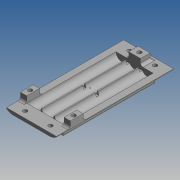
# Autodesk Inventor part: P040_BoitierCouvercleV4_module
Saved by Autodesk Inventor 2021.3 (Build 253353000, 353)
## iProperties
Created: 2021-12-17
Part Number: P040_BoitierCouvercleV4_module
Material: Générique
Document SubType Name: Modeling
Designer: gabri
Density: 1 g/cm^3
Appearance: Par défaut
Author: gabri
Autodesk Inventor part; units mm, degrees
note: some values were not read from the file. Chosen so that the rebuilt part matches the saved one: direction of "Hole1".
ref_plane "YZ Plane" through (0, 0, 0) normal (1, 0, 0) x (0, 1, 0)
ref_plane "XZ Plane" through (0, 0, 0) normal (0, 1, 0) x (-1, 0, 0)
sketch "Sketch2" plane through (0, 0, 0) normal (0, 0, 1) x (1, 0, 0)
  line L0 (30, -92) -> (-30, -92)
  line L1 (-30, -92) -> (-30, 92)
  line L2 (-30, 92) -> (30, 92)
  line L3 (30, 92) -> (30, -92)
  line L4 (30, -92) -> (-30, 92) construction
  line L5 (-30, -92) -> (30, 92) construction
  point P0 (0, 0)
  dimension "d0" = 60
  dimension "d1" = 184
  constraints: 12 end point, 2 midpoint, 2 parallel, 1 horizontal, 1 perpendicular
  measures "d0" distance between parallel lines of L3 L1
  measures "d1" distance between parallel lines of L0 L2
extrude "Extrusion1" add sketch "Sketch2" along normal blind 5
sketch "Sketch3" plane through (0, 0, 5) normal (0, 0, 1) x (1, 0, 0)
  line L0 (-30, -92) -> (30, -92) construction
  line L1 (30, 92) -> (-30, 92) construction
  line L2 (30, -92) -> (30, 92) construction
  line L3 (-30, 92) -> (-30, -92) construction
  point P0 (0, 0)
  point P1 (-20, 82)
  point P2 (20, 82)
  point P3 (-20, -82)
  point P4 (20, -82)
  dimension "d4" = 40
  dimension "d5" = 164
  dimension "d6" = 184
  dimension "d7" = 60
  dimension "d8" = 10
  dimension "d9" = 10
  dimension "d10" = 10
  dimension "d11" = 164
  dimension "d12" = 40
  dimension "d13" = 10
  measures "d4" distance of point (20, 82) point (-20, 82)
  measures "d5" distance of point (-20, 82) point (-20, -82)
  measures "d6" distance between parallel lines of L0 L1
  measures "d7" distance between parallel lines of L2 L3
  measures "d8" distance from line of L3 point (-20, 82)
  measures "d9" distance from line of L1 point (-20, 82)
  measures "d10" distance from line of L1 point (20, 82)
  measures "d11" distance of point (20, -82) point (20, 82)
  measures "d12" distance of point (20, -82) point (-20, -82)
  measures "d13" distance from line of L3 point (-20, -82)
hole "Hole1" at (-20, 82, 5) at (20, 82, 5) at (-20, -82, 5) at (20, -82, 5) direction (0, 0, -1) diameter 6.4 depth 5
sketch "Sketch4" plane through (0, 0, 5) normal (0, 0, 1) x (1, 0, 0)
  line L0 (-13.7576, 88.5859) -> (-6.8739, 88.5859) construction
  line L1 (-6.8739, 88.5859) -> (-6.8739, 84.2378) construction
  line L2 (-6.8739, 84.2378) -> (-13.7576, 84.2378) construction
  line L3 (-13.7576, 84.2378) -> (-13.7576, 88.5859) construction
  point P0 (0, 0)
  constraints: 2 other
sketch "Sketch5" plane through (0, 0, 5) normal (0, 0, 1) x (1, 0, 0)
  line L0 (-30, -72) -> (30, -72)
  line L1 (30, -72) -> (30, 72)
  line L2 (30, 72) -> (-30, 72)
  line L3 (-30, 72) -> (-30, -72)
  line L4 (-30, -72) -> (30, 72) construction
  line L5 (30, -72) -> (-30, 72) construction
  circle A0 centre (-20, -82) radius 3.2 construction
  circle A1 centre (-20, 82) radius 3.2 construction
  circle A2 centre (20, 82) radius 3.2 construction
  circle A3 centre (20, -82) radius 3.2 construction
  line L6 (30, 92) -> (-30, 92) construction
  line L7 (-30, 92) -> (-30, -92) construction
  line L8 (-30, -92) -> (30, -92) construction
  line L9 (30, -92) -> (30, 92) construction
  point P0 (0, 0)
  point P1 (30, 0)
  dimension "d21" = 10
  constraints: 12 end point, 4 midpoint, 2 parallel, 1 horizontal, 1 perpendicular
  measures "d21" distance from line of A2.centre L2
extrude "Extrusion2" add sketch "Sketch5" against normal blind 15
sketch "Sketch6" plane through (0, 0, 0) normal (0, 1, 0) x (-1, 0, 0)
  line L0 (-30, 5) -> (30, 5) construction
  line L1 (30, -10) -> (-30, -10) construction
  line L2 (30, 0) -> (30, 5) construction
  line L3 (-30, 0) -> (-30, 5) construction
  circle A0 centre (0, 5) radius 9.25
  circle A1 centre (-20, 5) radius 9.25
  line L4 (0, -13.85) -> (0, 20.1) construction
  circle A2 centre (20, 5) radius 9.25
  point P0 (0, 0)
  dimension "d24" = 18.5
  dimension "d27" = 18.5
  dimension "d40" = 18.5
  dimension "d41" = 20
  dimension "d42" = 20
  constraints: 4 point on line, 3 centre point, 2 midpoint
  measures "d24" diameter of A0
  measures "d27" diameter of A1
  measures "d40" diameter of A2
  measures "d41" distance of A0.centre A2.centre
  measures "d42" distance from line of L4 A1.centre
extrude "Extrusion3" cut sketch "Sketch6" along normal mid plane 140
fillet "Fillet2" radius 6 2 edges at (0, 72, 0) (0, -72, 0)
ref_plane "Work Plane1" through (0, 0, 4) normal (0, 0, -1) x (-1, 0, 0)
sketch "Sketch9" plane through (0, 0, 4) normal (0, 0, -1) x (-1, 0, 0)
  line L0 (30, -72) -> (30, 72) construction
  line L1 (30, 78) -> (-30, 78) construction
  line L2 (30, 92) -> (30, 78) construction
  line L3 (-30, 92) -> (30, 92) construction
  line L4 (-30, 78) -> (-30, 92) construction
  circle A0 centre (20, 82) radius 3.2 construction
  circle A1 centre (-20, 82) radius 3.2 construction
  line L5 (-30, 78) -> (-30, 72) construction
  line L6 (-30, 72) -> (30, 72) construction
  line L7 (30, 72) -> (30, 78) construction
  line L8 (30, 78) -> (-30, 78) construction
  line L9 (-30, -78) -> (30, -78) construction
  line L10 (-30, -92) -> (-30, -78) construction
  line L11 (30, -92) -> (-30, -92) construction
  line L12 (30, -78) -> (30, -92) construction
  circle A2 centre (20, -82) radius 3.2 construction
  circle A3 centre (-20, -82) radius 3.2 construction
  line L13 (30, -72) -> (-30, -72) construction
  line L14 (30, -78) -> (30, -72) construction
  line L15 (30, -72) -> (-30, -72) construction
  line L16 (-30, -72) -> (-30, -78) construction
  line L17 (-30, -78) -> (30, -78) construction
  line L18 (-30, 92) -> (-39.25, 92)
  line L19 (-39.25, 92) -> (-39.25, -92)
  line L20 (-39.25, -92) -> (-30, -92)
  line L21 (-30, -92) -> (-30, 92)
  line L22 (30, 92) -> (39.25, 92)
  line L23 (39.25, 92) -> (39.25, -92)
  line L24 (39.25, -92) -> (30, -92)
  line L25 (30, -92) -> (30, 92)
  point P0 (0, 0)
  dimension "d44" = 9.25
  dimension "d45" = 184
  dimension "d46" = 9.25
  dimension "d47" = 184
  constraints: 16 end point, 4 parallel, 2 horizontal, 2 perpendicular
  measures "d44" distance between parallel lines of L4 L19
  measures "d45" distance between parallel lines of L20 L18
  measures "d46" distance between parallel lines of L23 L2
  measures "d47" distance between parallel lines of L22 L24
extrude "Extrusion5" add sketch "Sketch9" against normal blind 1
sketch "Sketch10" plane through (0, 0, 5) normal (0, 0, 1) x (1, 0, 0)
  line L0 (9.25, -70) -> (-9.25, -70) construction
  line L1 (-9.25, -70) -> (-9.25, 70) construction
  line L2 (-9.25, 70) -> (9.25, 70) construction
  line L3 (9.25, 70) -> (9.25, -70) construction
  line L4 (29.25, -70) -> (10.75, -70) construction
  line L5 (10.75, -70) -> (10.75, 70) construction
  line L6 (10.75, 70) -> (29.25, 70) construction
  line L7 (29.25, 70) -> (29.25, -70) construction
  line L8 (-10.75, -70) -> (-29.25, -70) construction
  line L9 (-29.25, -70) -> (-29.25, 70) construction
  line L10 (-29.25, 70) -> (-10.75, 70) construction
  line L11 (-10.75, 70) -> (-10.75, -70) construction
  circle A0 centre (20, -82) radius 3.2 construction
  circle A1 centre (-20, -82) radius 3.2 construction
  line L12 (39.25, 92) -> (-39.25, 92) construction
  line L13 (-39.25, 92) -> (-39.25, -92) construction
  line L14 (-39.25, -92) -> (39.25, -92) construction
  line L15 (39.25, -92) -> (39.25, 92) construction
  circle A2 centre (20, 82) radius 3.2 construction
  circle A3 centre (-20, 82) radius 3.2 construction
  line L16 (29.25, -70) -> (39.25, -70)
  line L17 (39.25, -70) -> (39.25, -50)
  line L18 (39.25, -50) -> (29.25, -50)
  line L19 (29.25, -50) -> (29.25, -70)
  line L20 (-29.25, -70) -> (-39.25, -70)
  line L21 (-39.25, -70) -> (-39.25, -50)
  line L22 (-39.25, -50) -> (-29.25, -50)
  line L23 (-29.25, -50) -> (-29.25, -70)
  line L24 (9.25, 85) -> (-9.25, 85)
  line L25 (-9.25, 85) -> (-9.25, 70)
  line L26 (-9.25, 70) -> (9.25, 70)
  line L27 (9.25, 70) -> (9.25, 85)
  point P0 (0, 0)
  dimension "d55" = 10
  dimension "d56" = 10
  dimension "d57" = 20
  dimension "d58" = 15
  dimension "d59" = 18.5
  constraints: 24 end point, 6 parallel, 3 horizontal, 3 perpendicular, 1 point on line
  measures "d55" distance between parallel lines of L7 L17
  measures "d56" distance between parallel lines of L21 L23
  measures "d57" distance between parallel lines of L16 L18
  measures "d58" distance between parallel lines of L2 L24
  measures "d59" distance between parallel lines of L25 L27
extrude "Extrusion6" add sketch "Sketch10" along normal blind 10
fillet "Fillet6" radius 4 7 edges at (34.25, -50, 5) (34.25, -70, 5) (-34.25, -70, 5) (-34.25, -50, 5) (9.25, 77.5, 5) (0, 85, 5) (-9.25, 77.5, 5)
sketch "Sketch11" plane through (-30, 92, 0) normal (0, 1, 0) x (1, 0, 0)
  line L0 (60, 0) -> (0, 0) construction
  line L1 (0, 0) -> (0, -4) construction
  line L2 (-9.25, -4) -> (0, -4) construction
  line L3 (-9.25, -4) -> (-9.25, -5) construction
  line L4 (69.25, -5) -> (-9.25, -5) construction
  line L5 (69.25, -4) -> (69.25, -5) construction
  line L6 (60, -4) -> (69.25, -4) construction
  line L7 (60, 0) -> (60, -4) construction
  line L8 (69.25, -4) -> (60, -4)
  line L9 (0, 0) -> (0, -4)
  line L10 (0, -4) -> (-9.25, -4)
  line L11 (60, -4) -> (60, 0)
  arc A0 (0, 0) -> (-9.25, -4) centre (0.9827, -14.9678) ccw
  arc A1 (69.25, -4) -> (60, 0) centre (56.9429, -19.765) ccw
  point P0 (30, 0)
  dimension "d68" = 15
  dimension "d69" = 20
  constraints: 8 end point, 4 point on circle, 3 collinear, 2 centre point, 1 perpendicular
  measures "d68" radius of A0
  measures "d69" radius of A1
extrude "Extrusion7" add sketch "Sketch11" against normal up to surface (184 mm away)
fillet "Fillet7" radius 2 4 edges at (0, 72, -10) (-30, 0, -10) (0, -72, -10) (30, 0, -10)
sketch "Sketch12" plane through (0, 0, 15) normal (0, 0, 1) x (1, 0, 0)
  line L0 (0, 128.8) -> (0, -128.8) construction
  line L1 (-9.25, 85) -> (-9.25, 70) construction
  line L2 (-9.25, 70) -> (9.25, 70) construction
  line L3 (9.25, 70) -> (9.25, 85) construction
  line L4 (9.25, 85) -> (-9.25, 85) construction
  line L5 (39.25, -70) -> (39.25, -50) construction
  line L6 (39.25, -50) -> (29.25, -50) construction
  line L7 (29.25, -50) -> (29.25, -70) construction
  line L8 (29.25, -70) -> (39.25, -70) construction
  line L9 (-29.25, -50) -> (-39.25, -50) construction
  line L10 (-39.25, -50) -> (-39.25, -70) construction
  line L11 (-39.25, -70) -> (-29.25, -70) construction
  line L12 (-29.25, -70) -> (-29.25, -50) construction
  point P0 (0, 0)
  point P1 (0, 77.5)
  point P2 (-34.25, -60)
  point P3 (34.25, -60)
  dimension "d70" = 9.25
  dimension "d71" = 7.5
  dimension "d102" = 5
  dimension "d103" = 5
  dimension "d104" = 10
  dimension "d105" = 10
  constraints: 1 point on line
  measures "d70" distance from line of L3 point (0, 77.5)
  measures "d71" distance from line of L2 point (0, 77.5)
  measures "d102" distance from line of L12 point (-34.25, -60)
  measures "d103" distance from line of L5 point (34.25, -60)
  measures "d104" distance from line of L11 point (-34.25, -60)
  measures "d105" distance from line of L8 point (34.25, -60)
hole "Hole2" at (0, 77.5, 15) at (34.25, -60, 15) at (-34.25, -60, 15) direction (0, 0, -1) diameter 6.4 depth 9.5
sketch "Sketch13" plane through (0, 0, 5) normal (0, 0, 1) x (1, 0, 0)
  line L0 (-29.25, -70) -> (-29.25, -46) construction
  line L1 (-29.25, -70) -> (-10.75, -70) construction
  line L2 (-10.75, 70) -> (-10.75, -70) construction
  line L3 (-10.75, 70) -> (-29.25, 70) construction
  line L4 (-29.25, -46) -> (-29.25, 70) construction
  line L5 (-9.25, -70) -> (-9.25, 70) construction
  line L6 (-9.25, -70) -> (9.25, -70) construction
  line L7 (9.25, 70) -> (9.25, -70) construction
  line L8 (9.25, 70) -> (-9.25, 70) construction
  line L9 (10.75, -70) -> (10.75, 70) construction
  line L10 (10.75, -70) -> (29.25, -70) construction
  line L11 (29.25, -46) -> (29.25, -70) construction
  line L12 (29.25, 70) -> (29.25, -46) construction
  line L13 (29.25, 70) -> (10.75, 70) construction
  line L14 (-12.75, -70) -> (-7.25, -70)
  line L15 (-7.25, -70) -> (-7.25, -66)
  line L16 (-7.25, -66) -> (-12.75, -66)
  line L17 (-12.75, -66) -> (-12.75, -70)
  line L18 (7.25, -66) -> (7.25, -70)
  line L19 (7.25, -70) -> (12.75, -70)
  line L20 (12.75, -66) -> (7.25, -66)
  line L21 (12.75, -70) -> (12.75, -66)
  line L22 (-12.75, 2) -> (-12.75, -2)
  line L23 (-12.75, -2) -> (-7.25, -2)
  line L24 (-7.25, 2) -> (-12.75, 2)
  line L25 (-7.25, -2) -> (-7.25, 2)
  line L26 (7.25, 2) -> (7.25, -2)
  line L27 (7.25, -2) -> (12.75, -2)
  line L28 (12.75, 2) -> (7.25, 2)
  line L29 (12.75, -2) -> (12.75, 2)
  line L30 (-12.75, 70) -> (-12.75, 66)
  line L31 (-12.75, 66) -> (-7.25, 66)
  line L32 (-7.25, 70) -> (-12.75, 70)
  line L33 (-7.25, 66) -> (-7.25, 70)
  line L34 (7.25, 70) -> (7.25, 66)
  line L35 (7.25, 66) -> (12.75, 66)
  line L36 (12.75, 70) -> (7.25, 70)
  line L37 (12.75, 66) -> (12.75, 70)
  point P0 (-9.25, -46)
  point P1 (9.25, -70)
  point P2 (9.25, 70)
  point P3 (10.75, 70)
  point P4 (10.75, -70)
  point P5 (30.75, 70)
  point P6 (30.75, -70)
  point P7 (49.25, -70)
  point P8 (49.25, -46)
  point P9 (49.25, 70)
  point P10 (-29.25, 22)
  point P11 (-29.25, -2)
  point P12 (-10.75, -2)
  point P13 (-10.75, 138)
  point P14 (-29.25, 138)
  point P15 (-9.25, 138)
  point P16 (-9.25, -2)
  point P17 (9.25, -2)
  point P18 (9.25, 138)
  point P19 (10.75, 138)
  point P20 (10.75, -2)
  point P21 (29.25, -2)
  point P22 (29.25, 22)
  point P23 (29.25, 138)
  point P24 (-9.25, 22)
  point P25 (-9.25, -2)
  point P26 (9.25, -2)
  point P27 (9.25, 138)
  point P28 (-9.25, 138)
  point P29 (10.75, 138)
  point P30 (10.75, -2)
  point P31 (29.25, -2)
  point P32 (29.25, 138)
  point P33 (30.75, 138)
  point P34 (30.75, -2)
  point P35 (49.25, -2)
  point P36 (49.25, 22)
  point P37 (49.25, 138)
  point P38 (-29.25, 90)
  point P39 (-29.25, 66)
  point P40 (-10.75, 66)
  point P41 (-10.75, 206)
  point P42 (-29.25, 206)
  point P43 (-9.25, 206)
  point P44 (-9.25, 66)
  point P45 (9.25, 66)
  point P46 (9.25, 206)
  point P47 (10.75, 206)
  point P48 (10.75, 66)
  point P49 (29.25, 66)
  point P50 (29.25, 90)
  point P51 (29.25, 206)
  point P52 (-9.25, 90)
  point P53 (-9.25, 66)
  point P54 (9.25, 66)
  point P55 (9.25, 206)
  point P56 (-9.25, 206)
  point P57 (10.75, 206)
  point P58 (10.75, 66)
  point P59 (29.25, 66)
  point P60 (29.25, 206)
  point P61 (30.75, 206)
  point P62 (30.75, 66)
  point P63 (49.25, 66)
  point P64 (49.25, 90)
  point P65 (49.25, 206)
  dimension "d87" = 2
  dimension "d88" = 2
  dimension "d89" = 4
  dimension "d92" = 20
  dimension "d95" = 68
  constraints: 48 end point, 2 horizontal, 2 parallel, 1 perpendicular, 1 point on line, 1 vertical, 110 other
  measures "d87" distance between parallel lines of L17 L2
  measures "d88" distance between parallel lines of L5 L15
  measures "d89" distance between parallel lines of L16 L14
  measures "d92" distance of L0.end point (-9.25, -46)
  measures "d95" distance of L0.end point (-29.25, 22)
extrude "Extrusion8" cut sketch "Sketch13" against normal blind 5
equation "\"d8\" = -0.5 * d4 + 0.5 * d7"
equation "\"d9\" = -0.5 * d5 + 0.5 * d6"
equation "\"d10\" = d9"
equation "\"d11\" = d5"
equation "\"d12\" = d4"
equation "\"d13\" = d8"
equation "\"d24\" = d40"
equation "\"d27\" = d24"
equation "\"d44\" = d46"
body "Solid1"
